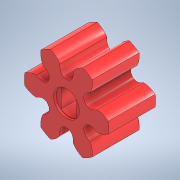
# Autodesk Inventor part: Linear pinion
Saved by Autodesk Inventor 2020 (Build 240168000, 168)
## iProperties
Created: 2021-06-18
Part Number: Linear pinion
Material: Generic
Document SubType Name: Modeling
Designer: ugwue
Density: 1 g/cm^3
Appearance: Light Red
Author: ugwue
Autodesk Inventor part; units mm, degrees
ref_plane "YZ Plane" through (0, 0, 0) normal (1, 0, 0) x (0, 1, 0)
ref_plane "XZ Plane" through (0, 0, 0) normal (0, 1, 0) x (-1, 0, 0)
ref_plane "XY Plane" through (0, 0, 0) normal (0, 0, 1) x (1, 0, 0)
sketch "Sketch1" plane through (0, 0, 0) normal (0, 0, 1) x (1, 0, 0)
  spline S0 degree 3 poles (-3.4392, 8.317) (-3.3361, 8.2682) (-3.1298, 8.1706) (-2.8322, 8.0009) (-2.5454, 7.8139) (-2.2723, 7.6072) (-2.0586, 7.4179) (-1.898, 7.2557) (-1.7835, 7.1285) (-1.6756, 6.9955) (-1.5762, 6.8563) (-1.4849, 6.7112) (-1.436, 6.608) (-1.4116, 6.5565) knots 0 0 0 0 0.034221 0.068441 0.102661 0.13688 0.171097 0.188208 0.20532 0.222431 0.239541 0.25665 0.273755 0.273755 0.273755 0.273755
  spline S1 degree 3 poles (-1.4116, 6.5565) (-1.4175, 6.497) (-1.4293, 6.3779) (-1.4313, 6.1984) (-1.4248, 6.0192) (-1.4058, 5.8406) (-1.3716, 5.6645) (-1.3259, 5.4908) (-1.2618, 5.3231) (-1.1833, 5.1616) (-1.0863, 5.0104) (-0.9725, 4.8713) (-0.8405, 4.7492) (-0.6925, 4.6469) (-0.5307, 4.5683) (-0.3583, 4.5166) (-0.1793, 4.4956) (0, 4.5022) (0.1793, 4.4956) (0.3583, 4.5166) (0.5307, 4.5683) (0.6925, 4.6469) (0.8405, 4.7492) (0.9725, 4.8713) (1.0863, 5.0104) (1.1833, 5.1616) (1.2618, 5.3231) (1.3259, 5.4908) (1.3716, 5.6645) (1.4058, 5.8406) (1.4248, 6.0192) (1.4313, 6.1984) (1.4293, 6.3779) (1.4175, 6.497) (1.4116, 6.5565) knots 0 0 0 0 0.017932 0.035866 0.053798 0.071731 0.089662 0.107593 0.125523 0.143448 0.16137 0.179295 0.197219 0.21514 0.23306 0.250976 0.26889 0.286823 0.304756 0.322671 0.340587 0.358507 0.376428 0.394352 0.412276 0.430199 0.448124 0.466054 0.483985 0.501916 0.519849 0.537781 0.555715 0.573647 0.573647 0.573647 0.573647
  spline S2 degree 3 poles (1.4116, 6.5565) (1.436, 6.608) (1.4849, 6.7112) (1.5762, 6.8563) (1.6756, 6.9955) (1.7835, 7.1285) (1.898, 7.2557) (2.0586, 7.4179) (2.2723, 7.6072) (2.5454, 7.8139) (2.8322, 8.0009) (3.1298, 8.1706) (3.3361, 8.2682) (3.4392, 8.317) knots 0 0 0 0 0.017105 0.034214 0.051324 0.068435 0.085546 0.102658 0.136875 0.171094 0.205314 0.239534 0.273755 0.273755 0.273755 0.273755
  circle A0 centre (0, 0) radius 4.5 construction
  circle A1 centre (0, 0) radius 6.5778 construction
  circle A2 centre (0, 0) radius 7 construction
  circle A3 centre (0, 0) radius 9
  point P0 (-3.1318, 8.1667)
  point P1 (-2.834, 7.998)
  point P2 (-2.5477, 7.8106)
  point P3 (-2.2751, 7.6038)
  point P4 (-2.0193, 7.3765)
  point P5 (-1.899, 7.2548)
  point P6 (-1.7846, 7.1276)
  point P7 (-1.677, 6.9945)
  point P8 (-1.5775, 6.8553)
  point P9 (-1.4879, 6.7096)
  point P10 (-1.4267, 6.3778)
  point P11 (-1.4299, 6.1985)
  point P12 (-1.4227, 6.0193)
  point P13 (-1.4033, 5.841)
  point P14 (-1.3697, 5.6649)
  point P15 (-1.3229, 5.4918)
  point P16 (-1.2594, 5.3241)
  point P17 (-1.1802, 5.1633)
  point P18 (-1.0835, 5.0124)
  point P19 (-0.9695, 4.8741)
  point P20 (-0.8378, 4.7525)
  point P21 (-0.6902, 4.6509)
  point P22 (-0.5289, 4.5728)
  point P23 (-0.3572, 4.5218)
  point P24 (-0.1793, 4.5002)
  point P25 (0, 4.5)
  point P26 (0.1793, 4.5002)
  point P27 (0.3572, 4.5218)
  point P28 (0.5289, 4.5728)
  point P29 (0.6902, 4.6509)
  point P30 (0.8378, 4.7525)
  point P31 (0.9695, 4.8741)
  point P32 (1.0835, 5.0124)
  point P33 (1.1802, 5.1633)
  point P34 (1.2594, 5.3241)
  point P35 (1.3229, 5.4918)
  point P36 (1.3697, 5.6649)
  point P37 (1.4033, 5.841)
  point P38 (1.4227, 6.0193)
  point P39 (1.4299, 6.1985)
  point P40 (1.4267, 6.3778)
  point P41 (1.4879, 6.7096)
  point P42 (1.5775, 6.8553)
  point P43 (1.677, 6.9945)
  point P44 (1.7846, 7.1276)
  point P45 (1.899, 7.2548)
  point P46 (2.0193, 7.3765)
  point P47 (2.2751, 7.6038)
  point P48 (2.5477, 7.8106)
  point P49 (2.834, 7.998)
  point P50 (3.1318, 8.1667)
  constraints: 4 centre point, 2 point on circle, 117 other
extrude "Extrusion1" add sketch "Sketch1" against normal blind 10
extrude "Extrusion2" cut sketch "Sketch1" against normal blind 10 contours A3 S2 S1 S0 picked at (0, 7.371)
pattern_circular "Circular Pattern1" count 6 over 360 about axis through (0, 0, 0) along (0, 0, -1) of "Extrusion2"
sketch "Sketch2" plane through (0, 0, 0) normal (0, 0, 1) x (1, 0, 0)
  line L0 (1.65, -2.0584) -> (1.65, 2.0584)
  line L1 (-1.65, 2.0584) -> (-1.65, -2.0584)
  line L2 (-1.65, -2.0584) -> (1.65, 2.0584) construction
  line L3 (1.65, -2.0584) -> (-1.65, 2.0584) construction
  arc A0 (-1.6689, -2.0584) -> (1.6689, -2.0584) centre (0, 0) ccw
  arc A1 (1.6574, 2.0677) -> (-1.6689, 2.0584) centre (0, 0) ccw
  line L4 (-1.65, 2.0584) -> (-1.65, 2.0736)
  line L5 (1.65, 2.0584) -> (1.65, 2.0736)
  line L6 (1.65, -2.0584) -> (1.65, -2.0736)
  line L7 (-1.65, -2.0736) -> (-1.65, -2.0584)
  dimension "d8" = 3.3
  constraints: 16 end point, 8 point on circle, 3 parallel, 2 centre point, 2 midpoint, 2 vertical, 1 coincident, 1 point on line
  measures "d8" distance of L1.end L0.start
extrude "Extrusion3" cut sketch "Sketch2" against normal blind 6
sketch "Sketch3" plane through (0, 0, 0) normal (0, 0, 1) x (1, 0, 0)
  circle A0 centre (0, 0) radius 2.75
  dimension "d11" = 5.5
  constraints: 1 centre point, 1 coincident
  measures "d11" diameter of A0
extrude "Extrusion4" cut sketch "Sketch3" against normal blind 0.5
equation "\"d0\" = FaceWidth"
equation "\"Module\" = 2"
equation "\"PressureAngle\" = 20deg"
equation "\"UnitProfileClearance\" = 0.25"
equation "\"UnitRoundRadius\" = 0.35"
equation "\"HeadDiameter\" = 18"
equation "\"RootDiameter\" = 9"
equation "\"BaseDiameter\" = 13.1557"
equation "\"PitchDiameter\" = 14"
equation "\"FaceWidth\" = 10"
equation "\"HelixAngle\" = 0"
equation "\"UnitCorrection\" = 0"
equation "\"UnitAddendumModification\" = 0"
equation "\"CircularPitch\" = 6.283185"
equation "\"UnitBacklashShift\" = 0"
equation "\"TotalToolShift\" = 0"
equation "\"IsInternal\" = 0"
body "Solid1"
